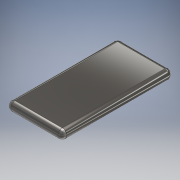
# Autodesk Inventor part: IphoneModel(Case)
Saved by Autodesk Inventor 2018 (Build 220112000, 112)
## iProperties
Created: 2017-07-25
Part Number: IphoneModel(Case)
Material: Generic
Document SubType Name: Modeling
Designer: kurtis
Density: 1 g/cm^3
Appearance: Steel - Polished
Author: kurtis
Autodesk Inventor part; units mm, degrees
ref_plane "YZ Plane" through (0, 0, 0) normal (1, 0, 0) x (0, 1, 0)
ref_plane "XZ Plane" through (0, 0, 0) normal (0, 1, 0) x (-1, 0, 0)
ref_plane "XY Plane" through (0, 0, 0) normal (0, 0, 1) x (1, 0, 0)
sketch "Sketch1" plane through (0, 0, 0) normal (0, 0, 1) x (1, 0, 0)
  line L0 (-36.5, -72.5) -> (36.5, -72.5)
  line L1 (36.5, -72.5) -> (36.5, 72.5)
  line L2 (36.5, 72.5) -> (-36.5, 72.5)
  line L3 (-36.5, 72.5) -> (-36.5, -72.5)
  line L4 (-36.5, -72.5) -> (36.5, 72.5) construction
  line L5 (36.5, -72.5) -> (-36.5, 72.5) construction
  point P0 (0, 0)
  dimension "d0" = 73
  dimension "d1" = 145
  constraints: 12 end point, 2 midpoint, 2 parallel, 1 horizontal, 1 perpendicular
  measures "d0" distance of L2.end L1.end
  measures "d1" distance of L1.end L0.end
extrude "Extrusion1" add sketch "Sketch1" along normal blind 12
fillet "Fillet1" radius 6 12 edges at (-36.5, 72.5, 6) (0, 72.5, 0) (0, 72.5, 12) (36.5, 72.5, 6) (36.5, 0, 0) (36.5, 0, 12) (-36.5, -72.5, 6) (0, -72.5, 0) (36.5, -72.5, 6) (0, -72.5, 12) (-36.5, 0, 12) (-36.5, 0, 0)
body "Solid1"
